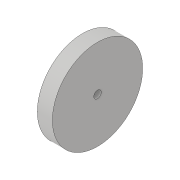
# Autodesk Inventor part: SUS-FrontWheel
Saved by Autodesk Inventor 2019.4 (Build 234330000, 330)
## iProperties
Created: 2020-02-24
Part Number: SUS-FrontWheel
Material: Generic
Document SubType Name: Modeling
Designer: Lord of Xy
Density: 1 g/cm^3
Appearance: Default
Author: Lord of Xy
Autodesk Inventor part; units mm, degrees
ref_plane "YZ Plane" through (0, 0, 0) normal (1, 0, 0) x (0, 1, 0)
ref_plane "XZ Plane" through (0, 0, 0) normal (0, 1, 0) x (-1, 0, 0)
ref_plane "XY Plane" through (0, 0, 0) normal (0, 0, 1) x (1, 0, 0)
sketch "Sketch2" plane through (0, 0, 0) normal (0, 1, 0) x (-1, 0, 0)
  line L0 (0, 6.35) -> (12.7, 6.35)
  line L1 (12.7, 6.35) -> (12.7, 76.2)
  line L2 (12.7, 76.2) -> (0, 76.2)
  line L3 (0, 76.2) -> (-12.7, 76.2)
  line L4 (-12.7, 76.2) -> (-12.7, 6.35)
  line L5 (-12.7, 6.35) -> (0, 6.35)
  line L6 (17.78, 0) -> (-17.78, 0) projected
  point P0 (0, 0)
  dimension "d0" = 76.2
  dimension "d1" = 25.4
  dimension "d2" = 6.35
  constraints: 12 end point, 3 perpendicular, 2 collinear, 1 horizontal, 1 point on line, 1 vertical, 1 vertical alignment
  measures "d0" distance from line of point (0, 0) L2
  measures "d1" distance between parallel lines of L4 L1
  measures "d2" distance from line of point (0, 0) L0
revolve "Revolution1" add sketch "Sketch2" angle 360 about axis through (-10, 0, 0) along (1, 0, 0)
body "Solid1"
